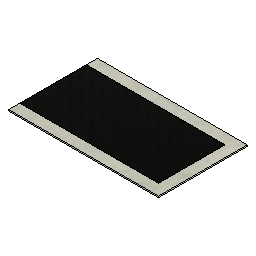
_End cap - Ruby.e0e99668-d129-415e-b873-1abbb96499f6 (Autodesk Fusion 360 design; units mm, degrees)
Autodesk Fusion 360 part; units mm, degrees
sketch "Sketch1" plane through (0, 0, 0) normal (0, 0, 1) x (1, 0, 0)
  line L0 (0, 0) -> (1270, 0)
  line L1 (1270, 0) -> (1270, -609.6)
  line L2 (1270, -609.6) -> (0, -609.6)
  line L3 (0, -609.6) -> (0, 0)
  dimension "d1" = 1270
  dimension "d2" = 609.6
  constraint horizontal L0
  constraint vertical L1
  constraint horizontal L2
  constraint vertical L3
  constraint coincident L0.start L3.end
  measures "d1" distance of L0.start L0.end
  measures "d2" distance of L0.start L2.end
extrude "Extrude1" add sketch "Sketch1" against normal blind 12.7 makes body 1
sketch "Sketch2" plane through (0, 0, 0) normal (0, 0, 1) x (-1, 0, 0)
  line L0 (0, 609.6) -> (-1270, 609.6)
  line L1 (-1270, 609.6) -> (-1270, 0)
  line L2 (-1270, 0) -> (0, 0)
  line L3 (0, 0) -> (0, 609.6)
  line L4 (0, 711.2) -> (-1371.6, 711.2)
  line L5 (-1371.6, 711.2) -> (-1371.6, -101.6)
  line L6 (-1371.6, -101.6) -> (0, -101.6)
  line L7 (0, -101.6) -> (0, 711.2)
  dimension "d5" = 101.6
  constraint perpendicular L4 L7
extrude "Extrude1'" add sketch "Sketch2" against normal blind 12.7 separate body contours L0 L1 L2 L4 L5 L6 L7 makes body 2 in component "Component"
copy_body "CutPasteBodies1" bodies 1 removing the originals makes body 3 in component "Component"
component "Component" placed x (1, 0, 0) y (0, 1, 0) z (0, 0, 1) at (0, 0, 0)
